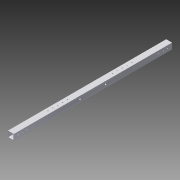
# Autodesk Inventor part: sidetube(st
Saved by Autodesk Inventor 2015 (Build 190159000, 159)
## iProperties
Created: 2015-09-27
Part Number: sidetube(st
Material: Aluminum 6061
Document SubType Name: Modeling
Designer: elilitwack
Density: 2.7 g/cm^3
Appearance: Aluminum - Flat
Mass: 381.427 g
Surface Area: 1791.19 cm^2
Volume: 141.269 cm^3
Author: elilitwack
Autodesk Inventor part; units mm, degrees
ref_plane "YZ Plane" through (0, 0, 0) normal (1, 0, 0) x (0, 1, 0)
ref_plane "XZ Plane" through (0, 0, 0) normal (0, 1, 0) x (-1, 0, 0)
ref_plane "XY Plane" through (0, 0, 0) normal (0, 0, 1) x (1, 0, 0)
sketch "profile_sketch" plane through (0, 0, 0) normal (0, 0, 1) x (1, 0, 0)
  line L0 (0, 0) -> (25.4, 0)
  line L1 (25.4, 0) -> (25.4, 25.4)
  line L2 (25.4, 25.4) -> (0, 25.4)
  line L3 (0, 25.4) -> (0, 0)
  line L4 (1.5875, 23.8125) -> (23.8125, 23.8125)
  line L5 (23.8125, 23.8125) -> (23.8125, 1.5875)
  line L6 (23.8125, 1.5875) -> (1.5875, 1.5875)
  line L7 (1.5875, 1.5875) -> (1.5875, 23.8125)
  dimension "d0" = 25.4
  dimension "d1" = 25.4
  dimension "d2" = 1.5875
  dimension "d3" = 1.5875
  dimension "d4" = 1.5875
  dimension "d5" = 1.5875
  constraints: 16 end point, 4 parallel, 2 horizontal, 2 perpendicular
  measures "d0" distance of L2.end L1.end
  measures "d1" distance of L1.end L0.end
  measures "d2" distance between parallel lines of L2 L4
  measures "d3" distance between parallel lines of L3 L7
  measures "d4" distance between parallel lines of L0 L6
  measures "d5" distance between parallel lines of L1 L5
extrude "profile_extrusion" add sketch "profile_sketch" along normal blind 685.8
sketch "gbmh_sketch" plane through (25.4, 0, 0) normal (1, 0, 0) x (0, 0, -1)
  line L0 (-685.8, 0) -> (-685.8, 25.4) construction
  line L1 (-685.8, 12.7) -> (-342.9, 12.7) construction
  line L2 (-342.9, 12.7) -> (0, 12.7) construction
  line L3 (0, 25.4) -> (0, 0) construction
  line L4 (-342.9, 12.7) -> (-342.9, 25.4) construction
  line L5 (0, 25.4) -> (-685.8, 25.4) construction
  line L6 (-342.9, 12.7) -> (-342.9, 0) construction
  point P0 (-398.4625, 12.7)
  point P1 (-287.3375, 12.7)
  dimension "d8" = 55.5752
  constraints: 8 end point, 3 midpoint, 2 collinear, 2 point on line, 1 horizontal, 1 symmetric about line
hole "gbmh" at (25.4, 12.7, 398.4625) at (25.4, 12.7, 287.3375) direction (-1, 0, 0) diameter 6.35 depth 25.4 tip angle 118
sketch "side_rivet_holes_sketch" plane through (0, 0, 0) normal (-1, 0, 0) x (0, 0, 1)
  line L0 (0, 25.4) -> (0, 0) construction
  line L1 (0, 12.7) -> (342.9, 12.7) construction
  line L2 (0, 1.5875) -> (685.8, 1.5875) construction
  line L3 (342.9, 12.7) -> (685.8, 12.7) construction
  line L4 (685.8, 25.4) -> (685.8, 0) construction
  line L5 (342.9, 12.7) -> (342.9, 25.4) construction
  line L6 (342.9, 12.7) -> (342.9, 0) construction
  line L7 (0, 0) -> (685.8, 0) construction
  point P0 (19.05, 12.7)
  point P1 (38.1, 12.7)
  point P2 (57.15, 12.7)
  point P3 (628.65, 12.7)
  point P4 (647.7, 12.7)
  point P5 (666.75, 12.7)
  dimension "d21" = 19.05
  dimension "d22" = 19.05
  dimension "d35" = 19.05
  dimension "d36" = 19.05
  dimension "d45" = 19.05
  dimension "d46" = 19.05
  constraints: 8 end point, 6 point on line, 3 midpoint, 2 collinear, 1 parallel, 1 vertical
  measures "d21" distance of point (38.1, 12.7) point (19.05, 12.7)
  measures "d22" distance of point (57.15, 12.7) point (38.1, 12.7)
  measures "d35" distance of point (647.7, 12.7) point (628.65, 12.7)
  measures "d36" distance of point (666.75, 12.7) point (647.7, 12.7)
  measures "d45" distance from line of L0 point (19.05, 12.7)
  measures "d46" distance from line of L4 point (666.75, 12.7)
hole "side_rivet_holes" at (0, 12.7, 19.05) at (0, 12.7, 38.1) at (0, 12.7, 57.15) at (0, 12.7, 628.65) at (0, 12.7, 647.7) at (0, 12.7, 666.75) direction (1, 0, 0) diameter 3.5719 depth 25.4 tip angle 118
sketch "crossbar_rivet_holes_sketch" plane through (0, 25.4, 0) normal (0, 1, 0) x (1, 0, 0)
  line L0 (0, 0) -> (0, -685.8) projected
  line L1 (25.4, 0) -> (25.4, -685.8) projected
  line L2 (25.4, -139.7) -> (0, -139.7) construction
  line L3 (25.4, -266.7) -> (0, -266.7) construction
  line L4 (25.4, -419.1) -> (0, -419.1) construction
  line L5 (0, 0) -> (0, -685.8) projected
  line L6 (25.4, -546.1) -> (0, -546.1) construction
  line L7 (25.4, 0) -> (0, 0) projected
  line L8 (25.4, -685.8) -> (0, -685.8) projected
  line L9 (12.7, -139.7) -> (12.7, -160.8667) construction
  line L10 (12.7, -160.8667) -> (12.7, -182.0333) construction
  line L11 (12.7, -182.0333) -> (12.7, -203.2) construction
  line L12 (12.7, -203.2) -> (12.7, -224.3667) construction
  line L13 (12.7, -224.3667) -> (12.7, -245.5333) construction
  line L14 (12.7, -245.5333) -> (12.7, -266.7) construction
  line L15 (12.7, -419.1) -> (12.7, -440.2667) construction
  line L16 (12.7, -440.2667) -> (12.7, -461.4333) construction
  line L17 (12.7, -461.4333) -> (12.7, -482.6) construction
  line L18 (12.7, -482.6) -> (12.7, -503.7667) construction
  line L19 (12.7, -503.7667) -> (12.7, -524.9333) construction
  line L20 (12.7, -524.9333) -> (12.7, -546.1) construction
  dimension "d48" = 127
  dimension "d49" = 127
  dimension "d52" = 203.2
  dimension "d53" = 203.2
  constraints: 32 end point, 15 point on line, 10 coincident, 10 collinear, 5 vertical, 4 midpoint, 4 perpendicular
  measures "d48" distance between parallel lines of L6 L4
  measures "d49" distance between parallel lines of L3 L2
  measures "d52" distance from line of L8 point (12.7, -482.6)
  measures "d53" distance from line of L7 point (12.7, -203.2)
hole "tb_rivet_holes" at (12.7, 25.4, 160.8667) at (12.7, 25.4, 182.0333) at (12.7, 25.4, 203.2) at (12.7, 25.4, 224.3667) at (12.7, 25.4, 245.5333) at (12.7, 25.4, 440.2667) at (12.7, 25.4, 461.4333) at (12.7, 25.4, 482.6) at (12.7, 25.4, 503.7667) at (12.7, 25.4, 524.9333) direction (0, -1, 0) diameter 3.5719 depth 25.4 tip angle 118
equation "\"d0\" = st_outer_diameter"
equation "\"d1\" = st_outer_diameter"
equation "\"d2\" = st_wall_thickness"
equation "\"d3\" = st_wall_thickness"
equation "\"d4\" = st_wall_thickness"
equation "\"d5\" = st_wall_thickness"
equation "\"d6\" = st_length"
equation "\"d14\" = gb_mh_diameter"
equation "\"d21\" = st_rivet_distance"
equation "\"d22\" = st_rivet_distance"
equation "\"d35\" = st_rivet_distance"
equation "\"d36\" = st_rivet_distance"
equation "\"d45\" = st_rivet_distance"
equation "\"d46\" = st_rivet_distance"
equation "\"d38\" = rv_hole_diameter"
equation "\"d48\" = tb_rivet_row_length"
equation "\"d49\" = tb_rivet_row_length"
equation "\"d52\" = st_cutout_depth_right"
equation "\"d53\" = st_cutout_depth_left"
equation "\"d54\" = rv_hole_diameter"
equation "\"gb_mh_seperation\" = 111.1504"
equation "\"st_outer_diameter\" = 25.4"
equation "\"st_inner_diameter\" = 6.35"
equation "\"st_wall_thickness\" = 1.5875"
equation "\"st_length\" = 685.8"
equation "\"st_gbmh_from_center\" = 0.5 * gb_mh_seperation"
equation "\"st_cutout_depth\" = 254"
equation "\"st_rivet_distance\" = 19.05"
equation "\"gb_mh_diameter\" = 6.35"
equation "\"rv_hole_diameter\" = 3.57187"
equation "\"st_cutout_depth_right\" = 203.2"
equation "\"st_cutout_depth_left\" = 203.2"
equation "\"gb_width\" = 127"
equation "\"gb_axle_from_edge\" = 38.1"
equation "\"gb_bearing_diameter\" = 28.575"
equation "\"gb_to_bottom_of_side_assembly\" = 4.7752"
equation "\"tb_rivet_row_length\" = 127"
equation "\"tb_metal_thickness\" = 3.048"
equation "\"tb_hm_mounting_slot_length\" = 40.64"
equation "\"gb_mh_seperation_alt\" = 111.125"
equation "\"gb_axle_from_edge_alt\" = 43.1546"
body "Solid1"
